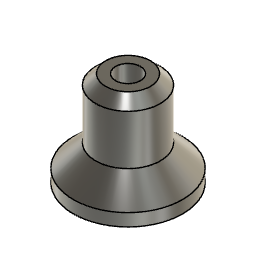
KitchenAid Mixer Feet (Autodesk Fusion 360 design; units mm, degrees)
Autodesk Fusion 360 part; units mm, degrees
note: some values were not read from the file. Set by a fixed rule: which sketch regions a step uses.
sketch "Base Revolution" plane through (0, 0, 0) normal (1, 0, 0) x (0, 1, 0)
  line L0 (0, 0) -> (0, 19) construction
  line L1 (0, 19) -> (2.5, 19) construction
  line L2 (2.5, 19) -> (4.5, 19)
  line L3 (4.5, 19) -> (6.5, 17)
  line L4 (6.5, 17) -> (6.5, 7)
  line L5 (6.5, 7) -> (11, 2.5)
  line L6 (11, 0) -> (2.5, 0)
  line L7 (2.5, 19) -> (2.5, 0)
  line L8 (11, 2.5) -> (11, 0)
  dimension "d2" = 12
  dimension "d3" = 19
  dimension "d4" = 4.5
  dimension "d5" = 6.5
  dimension "d6" = 2.5
  dimension "d7" = 135
  dimension "d8" = 135
  dimension "d10" = 8.5
  constraint coincident L0.start origin
  constraint vertical L0
  constraint perpendicular L0 L1
  constraint perpendicular L0 L2
  constraint vertical L7
  constraint vertical L4
  constraint coincident L0.start L6
  constraint horizontal L6
  constraint perpendicular L6 L8
  measures "d2" vertical distance of L2.end L4.end
  measures "d3" distance of L2.end L6
  measures "d4" distance of L0.end L2.end
  measures "d5" distance of L0 L3.end
  measures "d6" distance of L0.end L1.end
  measures "d7" angle of L4 L5
  measures "d8" angle of L2 L3
  measures "d10" distance of L6.end L6.start
revolve "Revolve1" add sketch "Base Revolution" angle 360 about axis through (0, 0, 0) along (0, 0, 1)
sketch "Foot cutout to reduce walking" plane through (0, 0, 0) normal (0, 1, 0) x (1, 0, 0)
  line L0 (11, -2.5) -> (-11, -2.5)
  line L1 (11, 0) -> (-11, 0)
  line L2 (2.5, 0) -> (-2.5, 0)
  line L3 (2.5, -19) -> (-2.5, -19)
  line L4 (8, 0) -> (7, -1)
  line L5 (7, -1) -> (6, 0)
  dimension "d11" = 3
  dimension "d14" = 2
  constraint coincident L1 L4.start
  constraint coincident L1 L5.end
  constraint equal L4 L5
  constraint perpendicular L4 L5
  measures "d11" distance of L1.start L4.start
  measures "d14" distance of L4.start L5.end
revolve "Revolve2" cut sketch "Foot cutout to reduce walking" angle 360 about axis through (0, 0, 1.75) along (0, 0, 1)
equation "d4 = ( 9 / 2 ) * 1 mm"
equation "d5 = ( 13 / 2 ) * 1 mm"
equation "d6 = ( 5 / 2 ) * 1 mm"
equation "d10 = ( 17 / 2 ) * 1 mm"
named bodies: "KitchenAid Mixer Feet"
